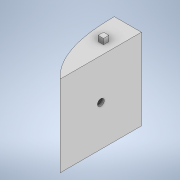
# Autodesk Inventor part: 3DPrintShapeStraightEdge1Simplified
Saved by Autodesk Inventor 2022 (Build 260153000, 153)
## iProperties
Created: 2022-04-20
Part Number: 3DPrintShapeStraightEdge1Simplified
Material: Generic
Document SubType Name: Modeling
Designer: Bruger
Density: 1 g/cm^3
Appearance: Default
Author: Bruger
Autodesk Inventor part; units mm, degrees
ref_plane "YZ Plane" through (0, 0, 0) normal (1, 0, 0) x (0, 1, 0)
ref_plane "XZ Plane" through (0, 0, 0) normal (0, 1, 0) x (-1, 0, 0)
ref_plane "XY Plane" through (0, 0, 0) normal (0, 0, 1) x (1, 0, 0)
sketch "Sketch1" plane through (0, 0, 0) normal (0, 1, 0) x (-1, 0, 0)
  line L0 (0, 0) -> (0, -150)
  line L1 (0, -150) -> (50, -150)
  line L2 (0, 0) -> (50, -44.9152) construction
  line L3 (50, -44.9152) -> (50, -150) construction
  spline S0 degree 2 poles (0, 0) (50, -44.9152) (50, -150) knots 1 1 1 2 2 2
  dimension "d0" = 150
  dimension "d2" = 50
  constraints: 4 end point, 1 horizontal, 1 vertical, 3 other
  measures "d0" distance of L0.start L0.end
  measures "d2" distance of L0.end L1.end
extrude "Extrusion7" add sketch "Sketch1" along normal blind 150
sketch "Sketch5" plane through (0, 0, -150) normal (0, 0, -1) x (-1, 0, 0)
  line L0 (0, 0) -> (0, 150) projected
  line L1 (0, 0) -> (20, 0)
  line L2 (0, 0) -> (50, 0) projected
  line L3 (20, 0) -> (20, 75)
  line L4 (25, 80) -> (15, 80)
  line L5 (15, 80) -> (15, 70)
  line L6 (15, 70) -> (25, 70)
  line L7 (25, 70) -> (25, 80)
  line L8 (25, 80) -> (15, 70) construction
  line L9 (15, 80) -> (25, 70) construction
  dimension "d57" = 20
  dimension "d58" = 75
  dimension "d59" = 10
  dimension "d60" = 10
  constraints: 16 end point, 2 midpoint, 2 parallel, 1 horizontal, 1 perpendicular, 1 point on line, 1 vertical
  measures "d57" distance of L0.start L1.end
  measures "d58" distance of L1.end L3.end
  measures "d59" distance of L6.end L5.end
  measures "d60" distance of L5.end L4.end
extrude "Extrusion8" add sketch "Sketch5" along normal blind 10
sketch "Sketch6" plane through (0, 0, 0) normal (0, -1, 0) x (1, 0, 0)
  line L0 (0, 0) -> (0, -150) projected
  line L1 (0, -150) -> (-20, -150)
  line L2 (0, -150) -> (-50, -150) projected
  line L3 (-20, -150) -> (-20, -100)
  line L4 (-25.15, -105.15) -> (-14.85, -105.15)
  line L5 (-14.85, -105.15) -> (-14.85, -94.85)
  line L6 (-14.85, -94.85) -> (-25.15, -94.85)
  line L7 (-25.15, -94.85) -> (-25.15, -105.15)
  line L8 (-25.15, -105.15) -> (-14.85, -94.85) construction
  line L9 (-14.85, -105.15) -> (-25.15, -94.85) construction
  dimension "d51" = 20
  dimension "d52" = 50
  dimension "d53" = 10.3
  dimension "d54" = 10.3
  constraints: 16 end point, 2 midpoint, 2 parallel, 2 perpendicular, 1 horizontal, 1 point on line
  measures "d51" distance of L0.end L1.end
  measures "d52" distance of L1.end L3.end
  measures "d53" distance of L6.end L5.end
  measures "d54" distance of L5.end L4.end
extrude "Extrusion9" cut sketch "Sketch6" against normal blind 10
sketch "Sketch7" plane through (0, 150, 0) normal (0, 1, 0) x (1, 0, 0)
  line L0 (0, 150) -> (-50, 150) projected
  line L1 (0, 150) -> (-20, 150)
  line L2 (-20, 150) -> (-20, 100)
  line L3 (-15, 95) -> (-25, 95)
  line L4 (-25, 95) -> (-25, 105)
  line L5 (-25, 105) -> (-15, 105)
  line L6 (-15, 105) -> (-15, 95)
  line L7 (-15, 95) -> (-25, 105) construction
  line L8 (-25, 95) -> (-15, 105) construction
  point P0 (0, 0)
  dimension "d61" = 20
  dimension "d62" = 50
  dimension "d63" = 10
  dimension "d64" = 10
  constraints: 16 end point, 2 midpoint, 2 parallel, 2 perpendicular, 1 horizontal, 1 point on line
  measures "d61" distance of L0.start L1.end
  measures "d62" distance of L1.end L2.end
  measures "d63" distance of L4.end L5.end
  measures "d64" distance of L3.end L4.end
extrude "Extrusion10" add sketch "Sketch7" along normal blind 10
sketch "Sketch8" plane through (0, 0, 0) normal (1, 0, 0) x (0, 0, -1)
  line L0 (0, 0) -> (0, 150) projected
  line L1 (0, 75) -> (75, 75) construction
  line L2 (0, 150) -> (150, 150) projected
  circle A0 centre (75, 75) radius 6.25
  line L3 (75, 75) -> (86, 75)
  line L4 (75, 75) -> (80.5, 84.5263)
  line L5 (75, 75) -> (69.5, 84.5263)
  line L6 (75, 75) -> (64, 75)
  line L7 (75, 75) -> (69.5, 65.4737)
  line L8 (75, 75) -> (80.5, 65.4737)
  line L9 (80.5, 65.4737) -> (86, 75)
  line L10 (80.5, 84.5263) -> (86, 75)
  line L11 (69.5, 84.5263) -> (80.5, 84.5263)
  line L12 (69.5, 84.5263) -> (64, 75)
  line L13 (64, 75) -> (69.5, 65.4737)
  line L14 (80.5, 65.4737) -> (69.5, 65.4737)
  dimension "d67" = 75
  dimension "d69" = 12.5
  dimension "d70" = 11
  dimension "d73" = 360
  constraints: 26 end point, 3 horizontal, 3 parallel, 1 centre point, 1 coincident, 1 midpoint, 1 point on line, 19 other
  measures "d67" distance of L1.start L1.end
  measures "d69" diameter of A0
  measures "d70" distance of L3.start L3.end
extrude "Extrusion11" cut sketch "Sketch8" against normal blind 100
extrude "Extrusion12" add sketch "Sketch8" against normal blind 5 contours L3 L9 L8 A0 | A0 L4 L10 L3 | A0 L5 L11 L4 | L8 L14 L7 A0 | A0 L6 L12 L5 | L7 L13 L6 A0
body "Solid2"
